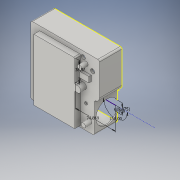
# Autodesk Inventor part: 01_Beamer_Gehäuse
Saved by Autodesk Inventor 2016 (Build 200138000, 138)
## iProperties
Created: 2016-07-23
Part Number: 01_Beamer_Gehäuse
Material: PC/ABS-Kunststoff
Document SubType Name: Modeling
Designer: Bene
Density: 0.357273 g/cm^3
Appearance: Weiß
Mass: 38.2104 g
Surface Area: 791.842 cm^2
Volume: 106.95 cm^3
Sending System: Autodesk Inventor 2017
Preprocessor: ST-DEVELOPER v16.5
Title: C:\Users\Bene\Dropbox\Dokumente\Optical Design\Beamerscope\Inventor\01_Beamer_Gehäuse.stp
Author: Bene
Autodesk Inventor part; units mm, degrees
ref_plane "YZ Plane" through (0, 0, 0) normal (1, 0, 0) x (0, 1, 0)
ref_plane "XZ Plane" through (0, 0, 0) normal (0, 1, 0) x (-1, 0, 0)
ref_plane "XY Plane" through (0, 0, 0) normal (0, 0, 1) x (1, 0, 0)
sketch "Skizze6" plane through (0, 0, 0) normal (0, 1, 0) x (-1, 0, 0)
  line L0 (64, -63) -> (-64, -63)
  line L1 (-64, -63) -> (-64, 63)
  line L2 (-64, 63) -> (64, 63)
  line L3 (64, 63) -> (64, -63)
  line L4 (64, -63) -> (-64, 63) construction
  line L5 (-64, -63) -> (64, 63) construction
  point P0 (0, 0)
  dimension "d22" = 128
  dimension "d23" = 126
  constraints: 12 end point, 2 midpoint, 2 parallel, 1 horizontal, 1 perpendicular
  measures "d22" distance of L1.end L2.end
  measures "d23" distance of L0.end L1.end
extrude "Extrusion5" add sketch "Skizze6" along normal blind 42
sketch "Skizze7" plane through (0, 42, 0) normal (0, 1, 0) x (1, 0, 0)
  line L0 (64, 63) -> (-64, 63) projected
  line L1 (-64, 63) -> (-64, -63) projected
  line L2 (-64, -63) -> (64, -63) projected
  line L3 (64, -63) -> (64, 63) projected
  line L4 (64, -63) -> (64, 63) projected
  line L5 (64, -63) -> (55, -63)
  line L6 (55, -63) -> (55, 6)
  line L7 (55, 6) -> (64, 6)
  line L8 (64, 6) -> (64, -63)
  line L9 (64, 63) -> (-64, 63) projected
  line L10 (64, 63) -> (55, 63)
  line L11 (55, 63) -> (55, 6)
  line L12 (55, 6) -> (64, 6)
  line L13 (64, 6) -> (64, 63)
  point P0 (0, 0)
  dimension "d26" = 9
  dimension "d27" = 69
  constraints: 16 end point, 4 parallel, 2 horizontal, 2 perpendicular
  measures "d26" distance of L6.end L7.end
  measures "d27" distance of L5.end L6.end
extrude "Extrusion6" cut sketch "Skizze7" against normal through all contours L3 L7 L11 L0
fillet "Rundung1" radius 8 1 edges at (64, 21, -6)
fillet "Rundung2" radius 3 5 edges at (64, 21, 63) (55, 21, -6) (55, 21, -63) (-64, 21, -63) (-64, 21, 63)
sketch "Skizze8" plane through (0, 42, 0) normal (0, 1, 0) x (1, 0, 0)
  arc A0 (-64, -60) -> (-61, -63) centre (-61, -60) ccw projected
  line L0 (-61, -63) -> (61, -63) projected
  arc A1 (61, -63) -> (64, -60) centre (61, -60) ccw projected
  line L1 (64, -60) -> (64, -2) projected
  arc A2 (64, -2) -> (57.4545, 5.8667) centre (56, -2) ccw projected
  arc A3 (55, 8.8167) -> (57.4545, 5.8667) centre (58, 8.8167) ccw projected
  line L2 (55, 8.8167) -> (55, 60) projected
  arc A4 (55, 60) -> (52, 63) centre (52, 60) ccw projected
  line L3 (52, 63) -> (-61, 63) projected
  arc A5 (-61, 63) -> (-64, 60) centre (-61, 60) ccw projected
  line L4 (-64, 60) -> (-64, -60) projected
  arc A6 (-62, -60) -> (-61, -61) centre (-61, -60) ccw
  line L5 (-61, -61) -> (61, -61)
  arc A7 (61, -61) -> (62, -60) centre (61, -60) ccw
  line L6 (62, -60) -> (62, -2)
  arc A8 (62, -2) -> (57.0909, 3.9) centre (56, -2) ccw
  arc A9 (53, 8.8167) -> (57.0909, 3.9) centre (58, 8.8167) ccw
  line L7 (53, 8.8167) -> (53, 60)
  arc A10 (53, 60) -> (52, 61) centre (52, 60) ccw
  line L8 (52, 61) -> (-61, 61)
  arc A11 (-61, 61) -> (-62, 60) centre (-61, 60) ccw
  line L9 (-62, 60) -> (-62, -60)
  point P0 (0, 0)
  dimension "d32" = 2
  constraints: 12 point on circle, 10 end point, 6 centre point, 10 other
  measures "d32" distance between parallel lines of L4 L9
extrude "Extrusion7" cut sketch "Skizze8" against normal blind 38 contours L9 A11 L8 A10 L7 A9 A8 L6 A7 L5 A6
sketch "Skizze9" plane through (55, 42, -8.8167) normal (1, 0, 0) x (0, 0, -1)
  circle A0 centre (27.6833, -18.5) radius 21
  line L0 (54.1833, -42) -> (54.1833, 0) projected
  line L1 (51.1833, -42) -> (0, -42) projected
  point P0 (-8.8167, -42)
  dimension "d35" = 42
  dimension "d36" = 26.5
  dimension "d37" = 23.5
  constraints: 1 centre point
  measures "d35" diameter of A0
  measures "d36" distance from line of A0.centre L0
  measures "d37" distance from line of A0.centre L1
extrude "Extrusion8" cut sketch "Skizze9" against normal blind 38
sketch "Skizze10" plane through (0, 4, 0) normal (0, 1, 0) x (1, 0, 0)
  arc A0 (-62, -60) -> (-61, -61) centre (-61, -60) ccw projected
  line L0 (61, -61) -> (-61, -61) projected
  arc A1 (61, -61) -> (62, -60) centre (61, -60) ccw projected
  line L1 (62, -2) -> (62, -60) projected
  arc A2 (62, -2) -> (57.0909, 3.9) centre (56, -2) ccw projected
  arc A3 (53, 8.8167) -> (57.0909, 3.9) centre (58, 8.8167) ccw projected
  line L2 (53, 60) -> (53, 44.2942) projected
  arc A4 (53, 60) -> (52, 61) centre (52, 60) ccw projected
  line L3 (-61, 61) -> (52, 61) projected
  arc A5 (-61, 61) -> (-62, 60) centre (-61, 60) ccw projected
  line L4 (-62, -60) -> (-62, 60) projected
  line L5 (-59.9014, -5) -> (2.0986, -5)
  line L6 (2.0986, -5) -> (2.0986, -2)
  line L7 (2.0986, -2) -> (-59.9014, -2)
  line L8 (-59.9014, -2) -> (-59.9014, -5)
  line L9 (53, 28.7058) -> (17, 28.7058) projected
  line L10 (17, 28.7058) -> (17, 44.2942) projected
  line L11 (17, 44.2942) -> (53, 44.2942) projected
  line L12 (53, 28.7058) -> (53, 8.8167) projected
  point P0 (0, 0)
  dimension "d40" = 62
  dimension "d41" = 3
  dimension "d42" = 56
  dimension "d43" = 63
  constraints: 8 end point, 2 parallel, 1 horizontal, 1 perpendicular
  measures "d40" distance of L7.end L6.end
  measures "d41" distance of L6.end L5.end
  measures "d42" distance between parallel lines of L0 L5
  measures "d43" distance between parallel lines of L3 L7
extrude "Extrusion9" add sketch "Skizze10" along normal blind 38 contours L8 L7 L6 L5
sketch "Skizze11" plane through (0, 4, 0) normal (0, 1, 0) x (1, 0, 0)
  line L0 (-59.9014, -5) -> (-59.9014, -2) projected
  line L1 (-59.9014, -2) -> (2.0986, -2) projected
  line L2 (2.0986, -2) -> (2.0986, -5) projected
  line L3 (2.0986, -5) -> (-59.9014, -5) projected
  arc A0 (-62, -60) -> (-61, -61) centre (-61, -60) ccw projected
  line L4 (61, -61) -> (-61, -61) projected
  arc A1 (61, -61) -> (62, -60) centre (61, -60) ccw projected
  line L5 (62, -2) -> (62, -60) projected
  arc A2 (62, -2) -> (57.0909, 3.9) centre (56, -2) ccw projected
  arc A3 (53, 8.8167) -> (57.0909, 3.9) centre (58, 8.8167) ccw projected
  line L6 (53, 60) -> (53, 44.2942) projected
  arc A4 (53, 60) -> (52, 61) centre (52, 60) ccw projected
  line L7 (-61, 61) -> (52, 61) projected
  arc A5 (-61, 61) -> (-62, 60) centre (-61, 60) ccw projected
  line L8 (-62, -60) -> (-62, 60) projected
  line L9 (-59.9014, -5) -> (-59.9014, -2) projected
  line L10 (-59.9014, -2) -> (2.0986, -2) projected
  line L11 (2.0986, -2) -> (2.0986, -5) projected
  line L12 (2.0986, -5) -> (-59.9014, -5) projected
  arc A6 (-62, -60) -> (-61, -61) centre (-61, -60) ccw projected
  line L13 (61, -61) -> (-61, -61) projected
  arc A7 (61, -61) -> (62, -60) centre (61, -60) ccw projected
  line L14 (62, -2) -> (62, -60) projected
  arc A8 (62, -2) -> (57.0909, 3.9) centre (56, -2) ccw projected
  arc A9 (53, 8.8167) -> (57.0909, 3.9) centre (58, 8.8167) ccw projected
  line L15 (53, 60) -> (53, 44.2942) projected
  arc A10 (53, 60) -> (52, 61) centre (52, 60) ccw projected
  line L16 (-61, 61) -> (52, 61) projected
  arc A11 (-61, 61) -> (-62, 60) centre (-61, 60) ccw projected
  line L17 (-62, -60) -> (-62, 60) projected
  line L18 (53, 28.7058) -> (17, 28.7058) projected
  line L19 (17, 28.7058) -> (17, 44.2942) projected
  line L20 (17, 44.2942) -> (53, 44.2942) projected
  line L21 (53, 28.7058) -> (53, 8.8167) projected
  line L22 (53, 28.7058) -> (17, 28.7058) projected
  line L23 (17, 28.7058) -> (17, 44.2942) projected
  line L24 (17, 44.2942) -> (53, 44.2942) projected
  line L25 (53, 28.7058) -> (53, 8.8167) projected
  line L26 (-50, 9.2096) -> (-1.2096, 58)
  line L27 (-1.2096, 58) -> (-1.9167, 58.7071)
  line L28 (-1.9167, 58.7071) -> (-50.7071, 9.9167)
  line L29 (-50.7071, 9.9167) -> (-50, 9.2096)
  line L30 (-50, 9.2096) -> (-1.9167, 58.7071) construction
  line L31 (-1.2096, 58) -> (-50.7071, 9.9167) construction
  line L32 (-50, 9.2096) -> (19, 9.2096) construction
  line L33 (-64, 60) -> (-64, -60) projected
  line L34 (52, 63) -> (-61, 63) projected
  point P0 (0, 0)
  point P1 (-25.9584, 33.9584)
  dimension "d107" = 69
  dimension "d108" = 45
  dimension "d109" = 1
  dimension "d111" = 14
  dimension "d112" = 5
  constraints: 14 end point, 2 midpoint, 2 parallel, 1 equal length, 1 horizontal, 1 perpendicular
  measures "d107" distance of L26.start L26.end
  measures "d108" angle of L32 L26
  measures "d109" distance of L27.end L26.end
  measures "d111" distance from line of L33 L26.start
  measures "d112" distance from line of L34 L26.end
extrude "Extrusion10" add sketch "Skizze11" along normal blind 38 contours L29 L28 L27 L26
sketch "Skizze12" plane through (0, 0, 0) normal (0, -1, 0) x (1, 0, 0)
  arc A0 (-61, 63) -> (-64, 60) centre (-61, 60) ccw construction
  line L0 (-64, 60) -> (-64, -60) construction
  arc A1 (-64, -60) -> (-61, -63) centre (-61, -60) ccw construction
  line L1 (-61, -63) -> (52, -63) construction
  arc A2 (52, -63) -> (55, -60) centre (52, -60) ccw construction
  line L2 (55, -60) -> (55, -8.8167) construction
  arc A3 (57.4545, -5.8667) -> (55, -8.8167) centre (58, -8.8167) ccw construction
  arc A4 (57.4545, -5.8667) -> (64, 2) centre (56, 2) ccw construction
  line L3 (64, 2) -> (64, 60) construction
  arc A5 (64, 60) -> (61, 63) centre (61, 60) ccw construction
  line L4 (61, 63) -> (-61, 63) construction
  line L5 (55, -63) -> (39.5, -63) construction
  line L6 (39.5, -63) -> (39.5, -5.8667) construction
  line L7 (39.5, -5.8667) -> (55, -5.8667) construction
  line L8 (55, -5.8667) -> (55, -63) construction
  circle A6 centre (39.5, -52) radius 1.5
  circle A7 centre (39.5, -18.5) radius 1.5
  point P0 (0, 0)
  dimension "d51" = 15.5
  dimension "d52" = 3
  dimension "d53" = 3
  dimension "d54" = 11
  dimension "d55" = 33.5
  constraints: 8 end point, 2 centre point, 2 parallel, 2 point on line, 1 horizontal, 1 perpendicular
  measures "d51" distance of L6.end L7.end
  measures "d52" diameter of A6
  measures "d53" diameter of A7
  measures "d54" distance of A6.centre L5.end
  measures "d55" distance of A7.centre A6.centre
extrude "Extrusion11" cut sketch "Skizze12" against normal blind 38
ref_plane "Arbeitsebene3" through (0, 5, 0) normal (0, 1, 0) x (1, 0, 0)
sketch "Skizze16" plane through (0, 0, 0) normal (0, -1, 0) x (1, 0, 0)
  circle A0 centre (46, -45) radius 4
  line L0 (-61, -63) -> (52, -63) projected
  line L1 (55, -60) -> (55, -8.8167) projected
  point P0 (0, 0)
  dimension "d66" = 8
  dimension "d67" = 18
  dimension "d68" = 9
  constraints: 1 centre point
  measures "d66" diameter of A0
  measures "d67" distance from line of A0.centre L0
  measures "d68" distance from line of A0.centre L1
extrude "Extrusion15" add sketch "Skizze16" along normal blind 12
sketch "Skizze17" plane through (0, 0, 0) normal (0, -1, 0) x (1, 0, 0)
  circle A0 centre (39.5, -18.5) radius 1.5 projected
  circle A1 centre (39.5, -52) radius 1.5 projected
  circle A2 centre (39.5, -18.5) radius 2.5
  circle A3 centre (39.5, -52) radius 2.5
  point P0 (0, 0)
  dimension "d71" = 1
  dimension "d72" = 1
  constraints: 2 centre point
  measures "d71" radial gap between concentric circles of A0 A2
  measures "d72" radial gap between concentric circles of A1 A3
extrude "Extrusion16" add sketch "Skizze17" along normal blind 1
sketch "Skizze18" plane through (0, 0, 0) normal (0, -1, 0) x (1, 0, 0)
  circle A0 centre (39.5, -18.5) radius 2.5 projected
  circle A1 centre (39.5, -52) radius 2.5 projected
  circle A2 centre (46, -45) radius 4 projected
  arc A3 (-61, 63) -> (-64, 60) centre (-61, 60) ccw projected
  line L0 (-64, 60) -> (-64, -60) projected
  arc A4 (-64, -60) -> (-61, -63) centre (-61, -60) ccw projected
  line L1 (-61, -63) -> (52, -63) projected
  arc A5 (52, -63) -> (55, -60) centre (52, -60) ccw projected
  line L2 (55, -60) -> (55, -8.8167) projected
  arc A6 (57.4545, -5.8667) -> (55, -8.8167) centre (58, -8.8167) ccw projected
  arc A7 (57.4545, -5.8667) -> (64, 2) centre (56, 2) ccw projected
  line L3 (64, 2) -> (64, 60) projected
  arc A8 (64, 60) -> (61, 63) centre (61, 60) ccw projected
  line L4 (61, 63) -> (-61, 63) projected
  circle A9 centre (51.5, 39) radius 3.9
  circle A10 centre (34, 53) radius 3.9
  circle A11 centre (33, 36) radius 3.9
  point P0 (0, 0)
  dimension "d75" = 7.8
  dimension "d76" = 12.5
  dimension "d77" = 24
  dimension "d78" = 7.8
  dimension "d79" = 30
  dimension "d80" = 10
  dimension "d81" = 7.8
  dimension "d83" = 31
  dimension "d97" = 27
  constraints: 3 centre point
  measures "d75" diameter of A9
  measures "d76" distance from line of A9.centre L3
  measures "d77" distance from line of L4 A9.centre
  measures "d78" diameter of A10
  measures "d79" distance from line of A10.centre L3
  measures "d80" distance from line of A10.centre L4
  measures "d81" diameter of A11
  measures "d83" distance from line of A11.centre L3
  measures "d97" distance from line of A11.centre L4
extrude "Extrusion17" cut sketch "Skizze18" against normal blind 10 contours A9 | A10 | A11
sketch "Skizze19" plane through (0, 0, 0) normal (0, -1, 0) x (1, 0, 0)
  circle A0 centre (34, 53) radius 3.9 projected
  circle A1 centre (51.5, 39) radius 3.9 projected
  circle A2 centre (33, 36) radius 3.9 projected
  circle A3 centre (39.5, -18.5) radius 2.5 projected
  circle A4 centre (39.5, -52) radius 2.5 projected
  circle A5 centre (46, -45) radius 4 projected
  arc A6 (-61, 63) -> (-64, 60) centre (-61, 60) ccw projected
  line L0 (-64, 60) -> (-64, -60) projected
  arc A7 (-64, -60) -> (-61, -63) centre (-61, -60) ccw projected
  line L1 (-61, -63) -> (52, -63) projected
  arc A8 (52, -63) -> (55, -60) centre (52, -60) ccw projected
  line L2 (55, -60) -> (55, -8.8167) projected
  arc A9 (57.4545, -5.8667) -> (55, -8.8167) centre (58, -8.8167) ccw projected
  arc A10 (57.4545, -5.8667) -> (64, 2) centre (56, 2) ccw projected
  line L3 (64, 2) -> (64, 60) projected
  arc A11 (64, 60) -> (61, 63) centre (61, 60) ccw projected
  line L4 (61, 63) -> (-61, 63) projected
  circle A12 centre (39, 45) radius 4
  point P0 (0, 0)
  dimension "d87" = 8
  dimension "d88" = 18
  dimension "d89" = 25
  constraints: 1 centre point
  measures "d87" diameter of A12
  measures "d88" distance from line of L4 A12.centre
  measures "d89" distance from line of A12.centre L3
extrude "Extrusion18" add sketch "Skizze19" along normal up to surface (12 mm away) contours A12
sketch "Skizze20" plane through (0, 0, 0) normal (0, -1, 0) x (1, 0, 0)
  circle A0 centre (39, 45) radius 4 projected
  circle A1 centre (34, 53) radius 3.9 projected
  circle A2 centre (51.5, 39) radius 3.9 projected
  circle A3 centre (33, 36) radius 3.9 projected
  circle A4 centre (39.5, -18.5) radius 2.5 projected
  circle A5 centre (39.5, -52) radius 2.5 projected
  circle A6 centre (46, -45) radius 4 projected
  arc A7 (-61, 63) -> (-64, 60) centre (-61, 60) ccw projected
  line L0 (-64, 60) -> (-64, -60) projected
  arc A8 (-64, -60) -> (-61, -63) centre (-61, -60) ccw projected
  line L1 (-61, -63) -> (52, -63) projected
  arc A9 (52, -63) -> (55, -60) centre (52, -60) ccw projected
  line L2 (55, -60) -> (55, -8.8167) projected
  arc A10 (57.4545, -5.8667) -> (55, -8.8167) centre (58, -8.8167) ccw projected
  arc A11 (57.4545, -5.8667) -> (64, 2) centre (56, 2) ccw projected
  line L3 (64, 2) -> (64, 60) projected
  arc A12 (64, 60) -> (61, 63) centre (61, 60) ccw projected
  line L4 (61, 63) -> (-61, 63) projected
  line L5 (49, 31.5) -> (29, 31.5)
  line L6 (29, 31.5) -> (29, 21)
  line L7 (29, 21) -> (49, 21)
  line L8 (49, 21) -> (49, 31.5)
  point P0 (0, 0)
  dimension "d92" = 15
  dimension "d93" = 10.5
  dimension "d94" = 31.5
  dimension "d98" = 35
  constraints: 8 end point, 2 parallel, 1 horizontal, 1 perpendicular
  measures "d92" distance between parallel lines of L8 L3
  measures "d93" distance between parallel lines of L7 L5
  measures "d94" distance between parallel lines of L5 L4
  measures "d98" distance between parallel lines of L6 L3
extrude "Extrusion19" add sketch "Skizze20" along normal blind 4.5 contours L8 L7 L6 L5
sketch "Skizze21" plane through (0, 0, 0) normal (0, -1, 0) x (1, 0, 0)
  line L0 (49, 31.5) -> (49, 21) projected
  line L1 (49, 21) -> (29, 21) projected
  line L2 (29, 21) -> (29, 31.5) projected
  line L3 (29, 31.5) -> (49, 31.5) projected
  circle A0 centre (39, 45) radius 4 projected
  circle A1 centre (34, 53) radius 3.9 projected
  circle A2 centre (51.5, 39) radius 3.9 projected
  circle A3 centre (33, 36) radius 3.9 projected
  circle A4 centre (39.5, -18.5) radius 2.5 projected
  circle A5 centre (39.5, -52) radius 2.5 projected
  circle A6 centre (46, -45) radius 4 projected
  arc A7 (-61, 63) -> (-64, 60) centre (-61, 60) ccw projected
  line L4 (-64, 60) -> (-64, -60) projected
  arc A8 (-64, -60) -> (-61, -63) centre (-61, -60) ccw projected
  line L5 (-61, -63) -> (52, -63) projected
  arc A9 (52, -63) -> (55, -60) centre (52, -60) ccw projected
  line L6 (55, -60) -> (55, -8.8167) projected
  arc A10 (57.4545, -5.8667) -> (55, -8.8167) centre (58, -8.8167) ccw projected
  arc A11 (57.4545, -5.8667) -> (64, 2) centre (56, 2) ccw projected
  line L7 (64, 2) -> (64, 60) projected
  arc A12 (64, 60) -> (61, 63) centre (61, 60) ccw projected
  line L8 (61, 63) -> (-61, 63) projected
  line L9 (29, 55) -> (-47.0364, 55)
  line L10 (-47.0364, 55) -> (-47.0364, -59.5)
  line L11 (-47.0364, -59.5) -> (29, -59.5)
  line L12 (29, -59.5) -> (29, 55)
  circle A13 centre (34, 7) radius 6
  line L13 (-1.2096, -58) -> (-50, -9.2096) construction
  line L14 (-50, -9.2096) -> (-1.2096, -58) construction
  line L15 (-47.0364, -59.5) -> (-14.9051, -59.5) construction
  line L16 (-47.0364, -59.5) -> (-14.9051, -59.5) construction
  line L17 (-14.9051, -59.5) -> (-50.7396, -23.6655) construction
  line L18 (-47.0364, 55) -> (-50.7071, 51.3293)
  line L19 (-47.0364, 55) -> (-41.8452, 55) construction
  line L20 (-1.9167, -58.7071) -> (-50.7071, -9.9167) projected
  line L21 (-50.7071, 51.3293) -> (-50.7071, -9.9167)
  line L22 (2.0986, 5) -> (-59.9014, 5) projected
  line L23 (-50.7071, -9.9167) -> (-1.1238, -59.5)
  line L24 (3.6715, -59.5) -> (-1.1238, -59.5)
  point P0 (0, 0)
  dimension "d99" = 0
  dimension "d100" = 8
  dimension "d101" = 12
  dimension "d102" = 56
  dimension "d103" = 30
  dimension "d113" = 3.5
  dimension "d114" = 180
  dimension "d115" = 135
  dimension "d116" = 135
  constraints: 24 end point, 3 horizontal, 2 collinear, 2 equal length, 2 parallel, 2 perpendicular, 2 point on line, 1 centre point
  measures "d99" distance between parallel lines of L12 L2
  measures "d100" distance between parallel lines of L8 L9
  measures "d101" diameter of A13
  measures "d102" distance from line of L8 A13.centre
  measures "d103" distance from line of A13.centre L7
  measures "d113" distance between parallel lines of L5 L11
  measures "d114" angle of L15 L16
  measures "d115" angle of L15 L17
  measures "d116" angle of L18 L19
extrude "Extrusion20" add sketch "Skizze21" along normal blind 11 contours L2 L12 A13 L11 L23 L20 L10 L9 | A13 L12 | L12 A13 | L20 L23 L11 L10
fillet "Rundung3" radius 2 3 edges at (29, -5.5, 10.3166) (29, -5.5, 55) (29, -5.5, 3.6834)
sketch "Skizze22" plane through (0, 4, 0) normal (0, 1, 0) x (1, 0, 0)
  arc A0 (27, -55) -> (29, -53) centre (27, -53) ccw projected
  line L0 (27, -55) -> (-47.0364, -55) projected
  line L1 (-47.0364, -55) -> (-47.0364, 59.5) projected
  line L2 (-47.0364, 59.5) -> (29, 59.5) projected
  line L3 (29, 59.5) -> (29, 0.4162) projected
  arc A1 (29, 0.4162) -> (31.75, -1.4379) centre (31, 0.4162) ccw projected
  arc A2 (31.75, -12.5621) -> (31.75, -1.4379) centre (34, -7) ccw projected
  arc A3 (31.75, -12.5621) -> (29, -14.4162) centre (31, -14.4162) ccw projected
  line L4 (29, -14.4162) -> (29, -53) projected
  line L5 (26.7408, 0.4162) -> (26.7408, 57.2408)
  line L6 (26.7408, 57.2408) -> (-44.7772, 57.2408)
  line L7 (-44.7772, 57.2408) -> (-44.7772, -52.7408)
  line L8 (-44.7772, -52.7408) -> (26.7408, -52.7408)
  line L9 (26.7408, -52.7408) -> (26.7408, -14.4162)
  arc A4 (32.5972, -10.4678) -> (26.7408, -14.4162) centre (31, -14.4162) ccw
  arc A5 (32.5972, -10.4678) -> (32.5972, -3.5322) centre (34, -7) ccw
  arc A6 (26.7408, 0.4162) -> (32.5972, -3.5322) centre (31, 0.4162) ccw
  circle A7 centre (34, -53) radius 3.9 projected
  circle A8 centre (51.5, -39) radius 3.9 projected
  circle A9 centre (33, -36) radius 3.9 projected
  circle A10 centre (39.5, 18.5) radius 1.5 projected
  circle A11 centre (39.5, 52) radius 1.5 projected
  line L10 (17, 28.7058) -> (17, 44.2942) projected
  line L11 (17, 44.2942) -> (53, 44.2942) projected
  line L12 (53, 60) -> (53, 44.2942) projected
  arc A12 (53, 60) -> (52, 61) centre (52, 60) ccw projected
  line L13 (-61, 61) -> (52, 61) projected
  arc A13 (-61, 61) -> (-62, 60) centre (-61, 60) ccw projected
  line L14 (-62, -60) -> (-62, 60) projected
  arc A14 (-62, -60) -> (-61, -61) centre (-61, -60) ccw projected
  line L15 (61, -61) -> (-61, -61) projected
  arc A15 (61, -61) -> (62, -60) centre (61, -60) ccw projected
  line L16 (62, -2) -> (62, -60) projected
  arc A16 (62, -2) -> (57.0909, 3.9) centre (56, -2) ccw projected
  arc A17 (53, 8.8167) -> (57.0909, 3.9) centre (58, 8.8167) ccw projected
  line L17 (53, 28.7058) -> (53, 8.8167) projected
  line L18 (53, 28.7058) -> (17, 28.7058) projected
  line L19 (-1.2096, 58) -> (-50, 9.2096) projected
  line L20 (-59.9014, -2) -> (2.0986, -2) projected
  line L21 (2.0986, -2) -> (2.0986, -5) projected
  line L22 (2.0986, -5) -> (-59.9014, -5) projected
  line L23 (-59.9014, -5) -> (-59.9014, -2) projected
  line L24 (-50, 9.2096) -> (-50.7071, 9.9167) projected
  line L25 (-50.7071, 9.9167) -> (-1.9167, 58.7071) projected
  line L26 (-1.9167, 58.7071) -> (-1.2096, 58) projected
  point P0 (0, 0)
  constraints: 10 end point, 6 point on circle, 3 centre point, 7 other
extrude "Extrusion21" cut sketch "Skizze22" against normal blind 11 contours L22 L21 L20 L7 L19 L6 L5 L11 L10 L18 A6 A5 A4 L9 L8 | L7 L20 L21 L22 | L7 L25 L6 L19 | L7 L6 L25 | L18 L10 L11 L5
sketch "Skizze23" plane through (0, -7, 0) normal (0, 1, 0) x (1, 0, 0)
  line L0 (11, 42.2123) -> (9, 42.2123)
  line L1 (9, 42.2123) -> (9, 30.2123)
  line L2 (9, 30.2123) -> (11, 30.2123)
  line L3 (11, 30.2123) -> (11, 42.2123)
  line L4 (11, 42.2123) -> (9, 30.2123) construction
  line L5 (9, 42.2123) -> (11, 30.2123) construction
  line L6 (55, 57.5) -> (55, 15.5) projected
  line L7 (26.7408, 44.2942) -> (26.7408, 28.7058) projected
  line L8 (53, 28.7058) -> (26.7408, 28.7058) projected
  line L9 (53, 26.5627) -> (53, 28.7058) projected
  line L10 (55, 26.5627) -> (53, 26.5627) projected
  line L11 (55, 46.4373) -> (55, 26.5627) projected
  line L12 (53, 46.4373) -> (55, 46.4373) projected
  line L13 (53, 44.2942) -> (53, 46.4373) projected
  line L14 (26.7408, 44.2942) -> (53, 44.2942) projected
  point P0 (0, 0)
  point P1 (10, 36.2123)
  dimension "d119" = 2
  dimension "d120" = 12
  dimension "d121" = 44
  constraints: 12 end point, 2 midpoint, 2 parallel, 1 horizontal, 1 perpendicular
  measures "d119" distance of L2.end L1.end
  measures "d120" distance of L1.end L0.end
  measures "d121" distance between parallel lines of L3 L6
extrude "Extrusion22" add sketch "Skizze23" along normal up to surface (11 mm away) contours L3 L2 L1 L0
sketch "Skizze24" plane through (0, 42, 0) normal (0, 1, 0) x (1, 0, 0)
  line L0 (55, 26.5627) -> (53, 26.5627) projected
  line L1 (53, 26.5627) -> (53, 8.8167) projected
  arc A0 (53, 8.8167) -> (57.0909, 3.9) centre (58, 8.8167) ccw projected
  arc A1 (62, -2) -> (57.0909, 3.9) centre (56, -2) ccw projected
  line L2 (62, -2) -> (62, -60) projected
  arc A2 (61, -61) -> (62, -60) centre (61, -60) ccw projected
  line L3 (61, -61) -> (-61, -61) projected
  arc A3 (-62, -60) -> (-61, -61) centre (-61, -60) ccw projected
  line L4 (-62, -60) -> (-62, 60) projected
  arc A4 (-61, 61) -> (-62, 60) centre (-61, 60) ccw projected
  line L5 (-61, 61) -> (52, 61) projected
  arc A5 (53, 60) -> (52, 61) centre (52, 60) ccw projected
  line L6 (53, 60) -> (53, 46.4373) projected
  line L7 (53, 46.4373) -> (55, 46.4373) projected
  line L8 (55, 46.4373) -> (55, 60) projected
  arc A6 (55, 60) -> (52, 63) centre (52, 60) ccw projected
  line L9 (52, 63) -> (-61, 63) projected
  arc A7 (-61, 63) -> (-64, 60) centre (-61, 60) ccw projected
  line L10 (-64, 60) -> (-64, -60) projected
  arc A8 (-64, -60) -> (-61, -63) centre (-61, -60) ccw projected
  line L11 (-61, -63) -> (61, -63) projected
  arc A9 (61, -63) -> (64, -60) centre (61, -60) ccw projected
  line L12 (64, -60) -> (64, -2) projected
  arc A10 (64, -2) -> (57.4545, 5.8667) centre (56, -2) ccw projected
  arc A11 (55, 8.8167) -> (57.4545, 5.8667) centre (58, 8.8167) ccw projected
  line L13 (55, 8.8167) -> (55, 26.5627) projected
  line L14 (52.1589, 36.4998) -> (-22.7098, 36.4998)
  line L15 (52.1589, 36.4998) -> (127.0275, 36.4998) construction
  line L16 (-50, 9.2096) -> (-1.2096, 58) projected
  line L17 (-22.7098, 36.4998) -> (-22.7098, -2)
  point P0 (0, 0)
  dimension "d124" = 19.8746
  dimension "d125" = 180
  dimension "d126" = 9.9375
  dimension "d127" = 38.4998
  dimension "d128" = 74.8687
  constraints: 6 end point, 1 collinear, 1 horizontal, 1 point on line, 1 vertical
  measures "d124" distance between parallel lines of L0 L7
  measures "d125" angle of L14 L15
  measures "d126" distance from line of L14.start L7
  measures "d127" distance of L14.end L17.end
  measures "d128" distance of L14.start L14.end
